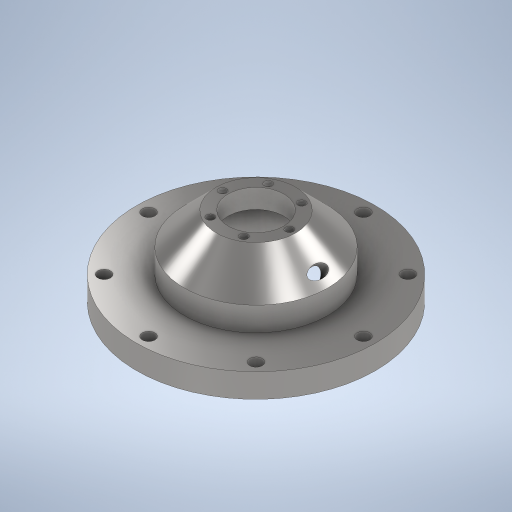
# Autodesk Inventor part: final injector body
Saved by Autodesk Inventor 2023 (Build 270158000, 158)
## iProperties
Created: 2022-09-20
Part Number: final injector body
Material: Stainless Steel
Document SubType Name: Modeling
Designer: pc
Density: 8 g/cm^3
Appearance: Semi-Polished
Author: pc
Autodesk Inventor part; units mm, degrees
ref_plane "XZ Plane" through (0, 0, 0) normal (0, 1, 0) x (-1, 0, 0)
ref_plane "XY Plane" through (0, 0, 0) normal (0, 0, 1) x (1, 0, 0)
sketch "Sketch1" plane through (0, 0, 0) normal (0, 0, 1) x (1, 0, 0)
  line L0 (0, 0) -> (0, 50)
  line L1 (45, 0) -> (75, 0)
  line L2 (75, 0) -> (75, 15)
  line L3 (75, 15) -> (45, 15)
  line L4 (45, 15) -> (45, 50)
  line L5 (45, 50) -> (0, 50)
  line L6 (0, 50) -> (0, 38)
  line L7 (45, 0) -> (45, 10)
  line L8 (45, 10) -> (35, 10)
  line L9 (35, 10) -> (35, 38)
  line L10 (35, 38) -> (0, 38)
  line L11 (0, 0) -> (35, 0)
  line L12 (45, 0) -> (45, 0)
  dimension "d1" = 50
  dimension "d2" = 15
  dimension "d4" = 12
  dimension "d5" = 10
  dimension "d6" = 150
  dimension "d7" = 90
  dimension "d8" = 70
  dimension "d9" = 10
  constraints: 26 end point, 5 perpendicular, 4 vertical, 3 point on line, 1 horizontal
  measures "d1" distance of L0.start L0.end
  measures "d2" distance of L1.end L2.end
  measures "d4" distance of L0.end L6.end
  measures "d5" distance of L1.start L7.end
  measures "d6" diameter of L2 L0
  measures "d7" diameter of L7 L0
  measures "d8" diameter of L9 L0
  measures "d9" distance between parallel lines of L4 L9
revolve "Revolution1" add sketch "Sketch1" angle 360 about axis through (0, 0, 0) along (0, 1, 0)
chamfer "Chamfer1" distance 20 angle 45 1 edges at (-45, 50, 0)
ref_plane "Work Plane1" through (45, 0, 0) normal (1, 0, 0) x (0, 1, 0)
sketch "Sketch4" plane through (45, 0, 0) normal (1, 0, 0) x (0, 1, 0)
  circle A0 centre (44.772, 0) radius 6.35
  point P0 (0, 0)
  dimension "d22" = 12.7
  constraints: 1 centre point
  measures "d22" diameter of A0
sketch "Sketch5" plane through (0, 0, 0) normal (0, 0, 1) x (1, 0, 0)
  line L0 (44.9751, 46.9317) -> (33.3301, 30)
  line L1 (45, 30) -> (-45, 30) projected
  point P0 (0, 0)
  constraints: 2 end point, 1 point on line
sweep "Sweep3" cut profiles "Sketch4" path "Sketch5" path curves L0
sketch "Sketch6" plane through (0, 50, 0) normal (0, 1, 0) x (1, 0, 0)
  circle A0 centre (0, 0) radius 17.5
  dimension "d25" = 35
  constraints: 1 centre point, 1 coincident
  measures "d25" diameter of A0
hole "Hole1" at (0, 50, 0) direction (0, -1, 0) diameter 35 depth 15 tip angle 118
sketch "Sketch7" plane through (0, 50, 0) normal (0, 1, 0) x (1, 0, 0)
  circle A0 centre (-21, 0) radius 2.75
  circle A1 centre (-10.5, -18.1865) radius 2.75
  circle A2 centre (10.5, -18.1865) radius 2.75
  circle A3 centre (21, 0) radius 2.75
  circle A4 centre (10.5, 18.1865) radius 2.75
  circle A5 centre (-10.5, 18.1865) radius 2.75
  point P0 (0, 0)
  dimension "d34" = 5.5
  dimension "d37" = 360
  dimension "d58" = 21
  constraints: 6 centre point, 13 other
  measures "d34" diameter of A0
  measures "d58" distance of A0.centre point (0, 0)
hole "Hole2" at (-10.5, 50, -18.1865) at (10.5, 50, -18.1865) at (21, 50, 0) at (10.5, 50, 18.1865) at (-10.5, 50, 18.1865) at (-21, 50, 0) direction (0, -1, 0) diameter 5 depth 10 tip angle 118
thread "Thread1"
thread "Thread2"
thread "Thread3"
thread "Thread4"
thread "Thread5"
thread "Thread6"
sketch "Sketch8" plane through (0, 15, 0) normal (0, 1, 0) x (1, 0, 0)
  point P0 (0, 0)
sketch "Sketch9" plane through (0, 0, 0) normal (0, -1, 0) x (1, 0, 0)
  point P0 (0, 0)
sketch "Sketch10" plane through (0, 0, 0) normal (0, -1, 0) x (1, 0, 0)
  point P0 (0, 0)
sketch "Sketch11" plane through (0, 0, 0) normal (0, -1, 0) x (1, 0, 0)
  circle A0 centre (0, 0) radius 17.5 projected
  circle A1 centre (0, 0) radius 67.5 construction
  circle A2 centre (67.5, 0) radius 4
  circle A3 centre (47.7297, -47.7297) radius 4
  circle A4 centre (0, -67.5) radius 4
  circle A5 centre (-47.7297, -47.7297) radius 4
  circle A6 centre (-67.5, 0) radius 4
  circle A7 centre (-47.7297, 47.7297) radius 4
  circle A8 centre (0, 67.5) radius 4
  circle A9 centre (47.7297, 47.7297) radius 4
  dimension "d59" = 135
  dimension "d60" = 8
  dimension "d94" = 360
  constraints: 8 centre point, 1 coincident, 1 horizontal alignment, 19 other
  measures "d60" diameter of A2
hole "Hole3" at (67.5, 0, 0) direction (0, 1, 0) diameter 8 end through all
hole "Hole4" at (47.7297, 0, 47.7297) at (0, 0, 67.5) at (-47.7297, 0, 47.7297) at (-67.5, 0, 0) at (-47.7297, 0, -47.7297) at (0, 0, -67.5) at (47.7297, 0, -47.7297) direction (0, 1, 0) diameter 8 end through all
body "Solid1"
